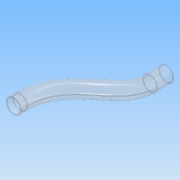
# Autodesk Inventor part: Top_End Pipe 3
Saved by Autodesk Inventor 2018.1 (Build 221171000, 171)
## iProperties
Created: 2019-03-21
Part Number: Top_End Pipe 3
Material: PMMA Plastic
Document SubType Name: Modeling
Designer: James
Density: 1.188 g/cm^3
Appearance: Polycarbonate - Clear
Author: James
Autodesk Inventor part; units mm, degrees
ref_plane "YZ Plane" through (0, 0, 0) normal (1, 0, 0) x (0, 1, 0)
ref_plane "XZ Plane" through (0, 0, 0) normal (0, 1, 0) x (-1, 0, 0)
ref_plane "XY Plane" through (0, 0, 0) normal (0, 0, 1) x (1, 0, 0)
sketch "Sketch1" plane through (0, 0, 0) normal (0, 1, 0) x (-1, 0, 0)
  circle A0 centre (0, 0) radius 23
  circle A1 centre (0, 0) radius 20
  dimension "d0" = 3
  dimension "d1" = 40
  constraints: 2 centre point, 2 coincident
  measures "d0" radial gap between concentric circles of A0 A1
  measures "d1" diameter of A1
extrude "Extrusion1" add sketch "Sketch1" along normal blind 50
sketch "Sketch2" plane through (0, 0, 0) normal (0, 0, 1) x (1, 0, 0)
  line L0 (23, 50) -> (-23, 50) projected
  point P0 (0, 0)
  point P1 (0, 43)
  point P2 (0, 50)
  dimension "d4" = 7
  constraints: 1 midpoint, 1 vertical alignment
  measures "d4" distance from line of L0 point (0, 43)
hole "Hole1" [suppressed]
sketch "Sketch3" plane through (0, 0, 0) normal (0, -1, 0) x (1, 0, 0)
  circle A0 centre (0, 0) radius 20 projected
  circle A1 centre (0, 0) radius 23 projected
sketch3d "3D Sketch1"
  spline S0 degree 3 poles (0, 0, 0) (0, -100, 0) (-150, -100, 0) (-150, -250, 0) knots 1 1 1 1 2 2 2 2
  dimension "d25" = 100
  dimension "d26" = 150
  dimension "d27" = 150
sweep "Sweep1" add profiles "Sketch3" path "3D Sketch1"
sketch "Sketch4" plane through (-150, -250, 0) normal (0, -1, 0) x (-1, 0, 0)
  spline S0 degree 6 poles (-20, 0) (-20, 33.2309) (21.091, 38.0022) (54.9823, 0) (21.091, -38.0022) (-20, -33.2309) (-20, 0) knots 0 0 0 0 0 0 0 1 1 1 1 1 1 1 weights 1.669078 1.03673 1.038347 0.853534 1.038347 1.03673 1.669078 projected
  circle A0 centre (0, 0) radius 23 projected
  point P0 (-150, 0)
  point P1 (-23, 0)
  constraints: 1 horizontal alignment, 1 other
extrude "Extrusion2" add sketch "Sketch4" along normal blind 20
body "Solid1"
